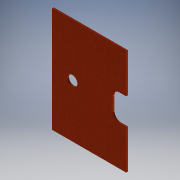
# Autodesk Inventor part: Back Panel Bottom
Saved by Autodesk Inventor 2016 (Build 200138000, 138)
## iProperties
Created: 2017-11-05
Part Number: Back Panel Bottom
Material: Generic
Document SubType Name: Modeling
Designer: mathaetaes
Density: 1 g/cm^3
Appearance: Default
Author: mathaetaes
Autodesk Inventor part; units mm, degrees
ref_plane "YZ Plane" through (0, 0, 0) normal (1, 0, 0) x (0, 1, 0)
ref_plane "XZ Plane" through (0, 0, 0) normal (0, 1, 0) x (-1, 0, 0)
ref_plane "XY Plane" through (0, 0, 0) normal (0, 0, 1) x (1, 0, 0)
sketch "Sketch1" plane through (0, 0, 0) normal (0, 0, 1) x (1, 0, 0)
  line L0 (-166.5857, -260.2376) -> (112.8143, -260.2376)
  line L1 (112.8143, -260.2376) -> (112.8143, 136.6374)
  line L2 (112.8143, 136.6374) -> (-166.5857, 136.6374)
  line L3 (-166.5857, 136.6374) -> (-166.5857, -260.2376)
  point P0 (0, 0)
  dimension "d0" = 396.875
  dimension "d3" = 279.4
  constraints: 8 end point, 2 parallel, 1 horizontal, 1 perpendicular
  measures "d0" distance of L2.end L0.start
  measures "d3" distance of L1.end L2.end
extrude "Board" add sketch "Sketch1" along normal blind 6.35
sketch "Sketch2" plane through (0, 0, 6.35) normal (0, 0, 1) x (1, 0, 0)
  circle A0 centre (-90.3857, -61.8001) radius 19.05
  line L0 (-166.5857, -260.2376) -> (112.8143, -260.2376) projected
  line L1 (-166.5857, 136.6374) -> (-166.5857, -260.2376) projected
  line L2 (112.8143, -260.2376) -> (112.8143, 136.6374) projected
  line L3 (112.8143, -112.6001) -> (87.4143, -112.6001)
  line L4 (62.0143, -87.2001) -> (62.0143, -36.4001)
  line L5 (87.4143, -11.0001) -> (112.8143, -11.0001)
  line L6 (112.8143, -11.0001) -> (112.8143, -112.6001)
  arc A1 (62.0143, -87.2001) -> (87.4143, -112.6001) centre (87.4143, -87.2001) ccw
  arc A2 (87.4143, -11.0001) -> (62.0143, -36.4001) centre (87.4143, -36.4001) ccw
  line L7 (112.8143, 136.6374) -> (-166.5857, 136.6374) projected
  point P0 (0, 0)
  point P1 (62.0143, -11.0001)
  dimension "d4" = 38.1
  dimension "d5" = 198.4375
  dimension "d6" = 76.2
  dimension "d9" = 50.8
  dimension "d10" = 25.4
  dimension "d11" = 101.6
  dimension "d12" = 25.4
  dimension "d13" = 147.6375
  constraints: 8 end point, 4 point on circle, 4 tangent, 3 centre point, 3 point on line, 2 parallel, 1 horizontal, 1 perpendicular
  measures "d4" diameter of A0
  measures "d5" distance from line of A0.centre L0
  measures "d6" distance from line of L1 A0.centre
  measures "d9" distance of point (62.014, -11) L5.end
  measures "d10" radius of A1
  measures "d11" distance between parallel lines of L5 L3
  measures "d12" radius of A2
  measures "d13" distance between parallel lines of L7 L5
extrude "Cutout Holes" cut sketch "Sketch2" against normal blind 6.35 contours A0 | L3 A1 L4 A2 L5 L2
equation "\"d5\" = 0.5 * d0"
equation "\"d13\" = -0.5 * d11 + 0.5 * d0"
body "Solid1"
